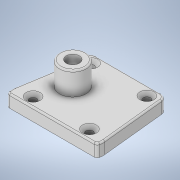
# Autodesk Inventor part: LegPin_Side_fillet_v1
Saved by Autodesk Inventor 2020.3 (Build 243373000, 373)
## iProperties
Created: 2021-03-02
Part Number: LegPin_Side_fillet_v1
Material: Generic
Document SubType Name: Modeling
Designer: sanyi
Density: 1 g/cm^3
Appearance: Default
Author: sanyi
Autodesk Inventor part; units mm, degrees
ref_plane "YZ Plane" through (0, 0, 0) normal (1, 0, 0) x (0, 1, 0)
ref_plane "XZ Plane" through (0, 0, 0) normal (0, 1, 0) x (-1, 0, 0)
ref_plane "XY Plane" through (0, 0, 0) normal (0, 0, 1) x (1, 0, 0)
sketch "Sketch1" plane through (0, 0, 0) normal (0, 1, 0) x (-1, 0, 0)
  line L0 (0, 114.579) -> (0, -115.31) construction
  line L1 (119.896, 0) -> (-136.2997, 0) construction
  line L2 (65, 45) -> (31.9074, 45) construction
  line L3 (-65, 45) -> (-65, 11.9074) construction
  line L4 (-65, -45) -> (-19.7, -45) construction
  line L5 (65, -45) -> (65, -11.9074) construction
  line L6 (64.9671, -36.1989) -> (82.3619, -53.5938) construction
  line L7 (82.3619, -53.5938) -> (73.5938, -62.3619) construction
  line L8 (73.5938, -62.3619) -> (56.1989, -44.9671) construction
  line L9 (56.1989, -44.9671) -> (64.9671, -36.1989) construction
  line L10 (64.9671, 36.1989) -> (82.3619, 53.5938) construction
  line L11 (82.3619, 53.5938) -> (73.5938, 62.3619) construction
  line L12 (73.5938, 62.3619) -> (56.1989, 44.9671) construction
  line L13 (56.1989, 44.9671) -> (64.9671, 36.1989) construction
  line L14 (-56.1989, 44.9671) -> (-73.5938, 62.3619) construction
  line L15 (-73.5938, 62.3619) -> (-82.3619, 53.5938) construction
  line L16 (-82.3619, 53.5938) -> (-64.9671, 36.1989) construction
  line L17 (-64.9671, 36.1989) -> (-56.1989, 44.9671) construction
  line L18 (-56.1989, -44.9671) -> (-73.5938, -62.3619) construction
  line L19 (-73.5938, -62.3619) -> (-82.3619, -53.5938) construction
  line L20 (-82.3619, -53.5938) -> (-64.9671, -36.1989) construction
  line L21 (-64.9671, -36.1989) -> (-56.1989, -44.9671) construction
  line L22 (55, 30) -> (-15, 30) construction
  line L23 (-15, 30) -> (-15, -30) construction
  line L24 (-15, -30) -> (55, -30) construction
  line L25 (55, -30) -> (55, 30) construction
  line L26 (73.6645, 44.8963) -> (64.8963, 53.6645) construction
  line L27 (68.7854, 57.5536) -> (77.5536, 48.7854) construction
  circle A0 centre (73.1695, 53.1695) radius 4.25 construction
  line L28 (73.6645, -44.8963) -> (64.8963, -53.6645) construction
  line L29 (77.5536, -48.7854) -> (68.7854, -57.5536) construction
  circle A1 centre (73.1695, -53.1695) radius 4.25 construction
  line L30 (-64.8963, 53.6645) -> (-73.6645, 44.8963) construction
  line L31 (-68.7854, 57.5536) -> (-77.5536, 48.7854) construction
  circle A2 centre (-73.1695, 53.1695) radius 4.25 construction
  line L32 (-73.6645, -44.8963) -> (-64.8963, -53.6645) construction
  line L33 (-77.5536, -48.7854) -> (-68.7854, -57.5536) construction
  circle A3 centre (-73.1695, -53.1695) radius 4.25 construction
  line L34 (6.8, 51.2) -> (-17.8, 51.2)
  line L35 (-17.8, 51.2) -> (-17.8, 38.8)
  line L36 (-17.8, 38.8) -> (6.8, 38.8)
  line L37 (6.8, 38.8) -> (6.8, 51.2)
  line L38 (6.8, -38.8) -> (-17.8, -38.8) construction
  line L39 (-17.8, -38.8) -> (-17.8, -51.2) construction
  line L40 (-17.8, -51.2) -> (6.8, -51.2) construction
  line L41 (6.8, -51.2) -> (6.8, -38.8) construction
  line L42 (6.8, 45) -> (-17.8, 45) construction
  line L43 (-5.5, 51.2) -> (-5.5, 38.8) construction
  line L44 (0, 51.2) -> (0, 38.8) construction
  line L45 (6.8, -45) -> (-17.8, -45) construction
  line L46 (-5.5, -38.8) -> (-5.5, -51.2) construction
  line L47 (0, -38.8) -> (0, -51.2) construction
  circle A4 centre (0, 45) radius 4.25
  circle A5 centre (0, -45) radius 4.25 construction
  line L48 (20, 30) -> (20, -30) construction
  line L49 (8.8, 57.2) -> (-19.8, 57.2)
  line L50 (8.8, -57.2) -> (-19.8, -57.2) construction
  line L51 (8.8, 57.2) -> (8.8, 45) construction
  line L52 (-19.8, 57.2) -> (-19.8, 45) construction
  line L53 (8.8, -57.2) -> (8.8, -45) construction
  line L54 (-19.8, -57.2) -> (-19.8, -45) construction
  line L55 (67.2298, 63.069) -> (61.3608, 57.2) construction
  line L56 (83.069, 47.2298) -> (77.2, 41.3608) construction
  line L57 (64.8963, 53.6645) -> (61.3608, 57.2) construction
  line L58 (73.6645, 44.8963) -> (77.2, 41.3608) construction
  arc A6 (83.069, 47.2298) -> (67.2298, 63.069) centre (75.1494, 55.1494) ccw construction
  line L59 (-61.3608, 57.2) -> (-67.2298, 63.069) construction
  line L60 (-83.069, 47.2298) -> (-77.2, 41.3608) construction
  line L61 (-61.3608, 57.2) -> (-64.8963, 53.6645) construction
  line L62 (-77.2, 41.3608) -> (-73.6645, 44.8963) construction
  arc A7 (-67.2298, 63.069) -> (-83.069, 47.2298) centre (-75.1494, 55.1494) ccw construction
  line L63 (73.6645, -44.8963) -> (77.2, -41.3608) construction
  line L64 (77.2, -41.3608) -> (83.069, -47.2298) construction
  line L65 (64.8963, -53.6645) -> (61.3608, -57.2) construction
  line L66 (61.3608, -57.2) -> (67.2298, -63.069) construction
  arc A8 (67.2298, -63.069) -> (83.069, -47.2298) centre (75.1494, -55.1494) ccw construction
  line L67 (-73.6645, -44.8963) -> (-77.2, -41.3608) construction
  line L68 (-64.8963, -53.6645) -> (-61.3608, -57.2) construction
  line L69 (-61.3608, -57.2) -> (-67.2298, -63.069) construction
  line L70 (-77.2, -41.3608) -> (-83.069, -47.2298) construction
  arc A9 (-83.069, -47.2298) -> (-67.2298, -63.069) centre (-75.1494, -55.1494) ccw construction
  arc A10 (23.5363, -45) -> (8.8, -57.2) centre (23.5363, -60) ccw construction
  arc A11 (61.3608, -57.2) -> (31.9074, -45) centre (31.9074, -86.6534) ccw construction
  arc A12 (65, -11.9074) -> (77.2, -41.3608) centre (106.6534, -11.9074) ccw construction
  arc A13 (77.2, 41.3608) -> (65, 11.9074) centre (106.6534, 11.9074) ccw construction
  arc A14 (31.9074, 45) -> (61.3608, 57.2) centre (31.9074, 86.6534) ccw construction
  arc A15 (8.8, 57.2) -> (23.5363, 45) centre (23.5363, 60) ccw
  arc A16 (-65, 11.9074) -> (-77.2, 41.3608) centre (-106.6534, 11.9074) ccw construction
  arc A17 (-77.2, -41.3608) -> (-65, -11.9074) centre (-106.6534, -11.9074) ccw construction
  line L71 (73.1695, -53.1695) -> (-73.1695, -53.1695) construction
  line L72 (-73.1695, 53.1695) -> (73.1695, 53.1695) construction
  line L73 (-61.3608, 57.2) -> (-61.3608, 45) construction
  line L74 (-61.3608, -57.2) -> (-61.3608, -45) construction
  arc A18 (-19.8, -57.2) -> (-34.5363, -45) centre (-34.5363, -60) ccw construction
  arc A19 (-31.9074, -45) -> (-61.3608, -57.2) centre (-31.9074, -86.6534) ccw construction
  arc A20 (-34.5363, 45) -> (-33.5506, 45.0324) centre (-34.5363, 60) ccw
  arc A21 (-61.3608, 57.2) -> (-33.5506, 45.0324) centre (-31.9074, 86.6534) ccw construction
  line L75 (73.5938, 62.3619) -> (76.4222, 65.1903) construction
  line L76 (76.4222, 65.1903) -> (85.1903, 56.4222) construction
  line L77 (85.1903, 56.4222) -> (82.3619, 53.5938) construction
  line L78 (79.3213, 59.3213) -> (59.2395, 39.2395) construction
  line L79 (59.2395, -39.2395) -> (79.3213, -59.3213) construction
  line L80 (-79.3213, 59.3213) -> (-59.2395, 39.2395) construction
  line L81 (-79.3213, -59.3213) -> (-59.2395, -39.2395) construction
  line L82 (75.1494, 55.1494) -> (77.9778, 57.9778) construction
  line L83 (75.1494, -55.1494) -> (77.9778, -57.9778) construction
  line L84 (-75.1494, -55.1494) -> (-77.9778, -57.9778) construction
  line L85 (-75.1494, 55.1494) -> (-77.9778, 57.9778) construction
  line L86 (-19.7, 45) -> (-65, 45) construction
  line L87 (8.7, 45) -> (-19.7, 45) construction
  line L88 (8.7, -45) -> (23.5363, -45) construction
  line L89 (-19.7, -45) -> (8.7, -45) construction
  line L90 (82.3619, 53.5938) -> (85.3751, 50.5805) construction
  line L91 (73.5938, 62.3619) -> (70.5805, 65.3751) construction
  line L92 (80.1698, 55.7858) -> (75.3615, 50.9775) construction
  line L93 (70.9775, -55.3615) -> (75.7858, -60.1698) construction
  line L94 (0, -48.1) -> (6.8, -48.1) construction
  line L95 (-75.3615, -50.9775) -> (-80.1698, -55.7858) construction
  line L96 (-75.7858, 60.1698) -> (-70.9775, 55.3615) construction
  line L97 (0, 48.1) -> (6.8, 48.1) construction
  line L98 (82.3619, -53.5938) -> (85.3751, -50.5805) construction
  line L99 (73.5938, -62.3619) -> (70.5805, -65.3751) construction
  line L100 (-73.5938, -62.3619) -> (-70.5805, -65.3751) construction
  line L101 (-82.3619, -53.5938) -> (-85.3751, -50.5805) construction
  line L102 (-73.5938, 62.3619) -> (-70.5805, 65.3751) construction
  line L103 (-82.3619, 53.5938) -> (-85.3751, 50.5805) construction
  line L104 (31.9074, 45) -> (23.5363, 45) construction
  line L105 (23.5363, 45) -> (8.7, 45) construction
  arc A22 (-33.5506, 45.0324) -> (-31.9074, 45) centre (-31.9074, 86.6534) ccw
  arc A23 (-33.5506, 45.0324) -> (-19.8, 57.2) centre (-34.5363, 60) ccw
  line L106 (-21.9995, 42) -> (-51.9995, 42) construction
  line L107 (-51.9995, 42) -> (-51.9995, -42) construction
  line L108 (-51.9995, -42) -> (-21.9995, -42) construction
  line L109 (-21.9995, -42) -> (-21.9995, 42) construction
  line L110 (52, 27) -> (55, 27) construction
  line L111 (52, -27) -> (55, -27) construction
  line L112 (52, 27) -> (52, 30) construction
  line L113 (-12, 27) -> (-12, 30) construction
  line L114 (-12, 27) -> (-15, 27) construction
  line L115 (-15, -27) -> (-12, -27) construction
  line L116 (-12, -27) -> (-12, -30) construction
  line L117 (52, -27) -> (52, -30) construction
  line L118 (-19.4995, 10) -> (-20.9995, 10) construction
  line L119 (-20.9995, 10) -> (-20.9995, -10) construction
  line L120 (-20.9995, -10) -> (-19.4995, -10) construction
  line L121 (-19.4995, -10) -> (-19.4995, 10) construction
  line L122 (-19.4995, 0) -> (-20.9995, 0) construction
  line L123 (-36.9995, 42) -> (-36.9995, -42) construction
  line L124 (-52.9995, 10) -> (-54.4995, 10) construction
  line L125 (-54.4995, 10) -> (-54.4995, -10) construction
  line L126 (-54.4995, -10) -> (-52.9995, -10) construction
  line L127 (-52.9995, -10) -> (-52.9995, 10) construction
  line L128 (-52.9995, 0) -> (-54.4995, 0) construction
  line L129 (31.9074, -45) -> (65, -45) construction
  line L130 (23.5363, -45) -> (31.9074, -45) construction
  line L131 (65, -11.9074) -> (65, 11.9074) construction
  line L132 (65, 11.9074) -> (65, 45) construction
  arc A24 (68.1707, 27.8475) -> (64.9671, 36.1989) centre (57.1958, 28.4277) ccw construction
  arc A25 (56.1989, 44.9671) -> (47.8475, 48.1707) centre (48.4277, 37.1958) ccw construction
  arc A26 (64.9671, -36.1989) -> (68.1707, -27.8475) centre (57.1958, -28.4277) ccw construction
  arc A27 (47.8475, -48.1707) -> (56.1989, -44.9671) centre (48.4277, -37.1958) ccw construction
  arc A28 (-56.1989, -44.9671) -> (-47.8475, -48.1707) centre (-48.4277, -37.1958) ccw construction
  arc A29 (-68.1707, -27.8475) -> (-64.9671, -36.1989) centre (-57.1958, -28.4277) ccw construction
  arc A30 (-48.6036, 48.4926) -> (-56.1989, 44.9671) centre (-47.5843, 36.3524) ccw construction
  arc A31 (-64.9671, 36.1989) -> (-68.1707, 27.8475) centre (-57.1958, 28.4277) ccw construction
  line L133 (-65, 11.9074) -> (-65, -11.9074) construction
  line L134 (-65, -11.9074) -> (-65, -45) construction
  line L135 (-56.1989, 44.9671) -> (-56.1989, -44.9671) construction
  arc A32 (-19.9504, 56.5) -> (-17.8, 51.2) centre (-15.1706, 55.3531) ccw
  arc A33 (6.8, 51.2) -> (8.9504, 56.5) centre (4.1706, 55.3531) ccw
  arc A34 (8.9504, -56.5) -> (6.8, -51.2) centre (4.1706, -55.3531) ccw construction
  arc A35 (-17.8, -51.2) -> (-19.9504, -56.5) centre (-15.1706, -55.3531) ccw construction
  line L136 (-17.8, 38.8) -> (-17.8, 32.8)
  line L137 (-17.8, 32.8) -> (6.8, 32.8)
  line L138 (6.8, 32.8) -> (6.8, 38.8)
  line L139 (-17.8, -38.8) -> (-17.8, -32.8) construction
  line L140 (-17.8, -32.8) -> (6.8, -32.8) construction
  line L141 (6.8, -32.8) -> (6.8, -38.8) construction
  line L142 (3.5, 54.2) -> (3.5, 35.8) construction
  line L143 (3.5, 35.8) -> (-14.5, 35.8) construction
  line L144 (-14.5, 35.8) -> (-14.5, 54.2) construction
  line L145 (-14.5, 54.2) -> (3.5, 54.2) construction
  line L146 (9.0232, 54.5696) -> (6.8, 40.8)
  line L147 (-20.0605, 54.8518) -> (-17.8, 32.8)
  point P0 (0, 0)
  point P1 (64.9853, 0)
  point P2 (55, 0)
  point P3 (60.583, -40.583)
  point P4 (-59.2395, 39.2395)
  point P5 (-60.583, 40.583)
  point P6 (-60.583, -40.583)
  point P7 (0, 45)
  point P8 (-33.9298, 45.0048)
  point P9 (-33.5506, -45.0324)
  point P10 (-56.1658, -45)
  point P11 (-56.2319, -45)
  point P12 (-56.2319, 45)
  point P13 (-56.1659, 45)
  point P14 (-20.0537, 54.7901)
  point P15 (6.8, 33.8)
  dimension "d0" = 135
  dimension "d4" = 24.6
  dimension "d5" = 12.4
  dimension "d6" = 70
  dimension "d7" = 60
  dimension "d9" = 8.5
  dimension "d10" = 135
  dimension "d12" = 6
  dimension "d13" = 2
  dimension "d14" = 2
  dimension "d16" = 20
  dimension "d23" = 5
  dimension "d29" = 130
  dimension "d32" = 15
  dimension "d33" = 4
  dimension "d34" = 28.4
  dimension "d38" = 4
  dimension "d40" = 6.8
  dimension "d49" = 30
  dimension "d50" = 84
  dimension "d51" = 3
  dimension "d52" = 3
  dimension "d53" = 1.5
  dimension "d54" = 20
  dimension "d59" = 1
  dimension "d60" = 90
  dimension "d61" = 135
  dimension "d70" = 135
  dimension "d82" = 0.7
  dimension "d83" = 0.7
  dimension "d84" = 0.7
  dimension "d85" = 0.7
  dimension "d86" = 6
  dimension "d102" = 18
  dimension "d126" = 2
  constraints: 294 end point, 89 tangent, 83 point on circle, 82 point on line, 80 perpendicular, 67 parallel, 42 midpoint, 40 equal length, 36 centre point, 18 horizontal, 15 collinear, 10 coincident, 8 equal radius, 7 symmetric about line, 3 vertical, 33 other
  measures "d0" angle of L3 L16
  measures "d4" distance between parallel lines of L11 L13
  measures "d5" distance between parallel lines of L10 L12
  measures "d6" distance of L24.end L23.end
  measures "d7" distance of L23.end L22.end
  measures "d9" diameter of A0
  measures "d10" angle of L6 L5
  measures "d12" distance between parallel lines of L34 L49
  measures "d13" distance between parallel lines of L37 L51
  measures "d14" distance between parallel lines of L41 L53
  measures "d16" distance between parallel lines of L0 L48
  measures "d23" distance between parallel lines of L56 L10
  measures "d29" distance between parallel lines of L3 L5
  measures "d32" radius of A15
  measures "d33" distance between parallel lines of L76 L11
  measures "d34" distance of L78.start L78.end
  measures "d38" distance of L82.start L82.end
  measures "d40" distance between parallel lines of L11 L27
  measures "d49" distance of L108.end L107.end
  measures "d50" distance of L107.end L106.end
  measures "d51" distance of L110.start L110.end
  measures "d52" distance of L110.start L112.end
  measures "d53" distance of L120.end L119.end
  measures "d54" distance of L119.end L118.end
  measures "d59" distance between parallel lines of L109 L119
  measures "d60" distance between parallel lines of L2 L88
  measures "d61" angle of L132 L10
  measures "d70" angle of L134 L20
  measures "d82" vertical distance of L49.end A32.start
  measures "d83" vertical distance of L49.start A33.end
  measures "d84" vertical distance of L50.start A34.start
  measures "d85" vertical distance of L50.end A35.end
  measures "d86" distance between parallel lines of L36 L137
  measures "d102" distance of L142.end L143.end
  measures "d126" distance from line of L36 L146.end
extrude "Extrusion12" add sketch "Sketch1" along normal blind 4 contours A33 L146 L37 | L34 A32 A23 L49 A15 A33 | L35 L136 L147 A32 | L36 L138 L137 L136
extrude "Extrusion13" add sketch "Sketch1" along normal blind 4 contours L37 L36 L35 L34
extrude "Extrusion14" add sketch "Sketch1" along normal blind 11.4 contours A4
sketch "Sketch2" plane through (0, 11.4, 45) normal (0, 1, 0) x (1, 0, 0)
  point P0 (0, 45)
  point P1 (0, 0)
hole "Hole3" at (0, 11.4, 45) direction (0, -1, 0) diameter 4.2 end through all
fillet "Fillet10" radius 2 2 edges at (-6.8, 2, 32.8) (17.8, 2, 32.8)
fillet "Fillet10" radius 1 2 edges at (19.8, 2, 57.2) (-8.8, 2, 57.2)
fillet "Fillet11" radius 0.5 11 edges at (19.6194, 4, 56.9798) (20.0778, 4, 55.6377) (-8.6194, 4, 56.9798) (-9.084, 4, 55.4955) (5.5, 4, 57.2) (5.5973, 4, 32.8) (4.25, 11.4, 45) (19.0223, 4, 44.7239) (17.3347, 4, 33.3154) (-6.2142, 4, 33.3858) (-7.9116, 4, 47.6848)
sketch "Sketch4" plane through (0, 4, 0) normal (0, 1, 0) x (1, 0, 0)
  point P0 (0, 0)
  point P1 (-3.5, -54.2)
  point P2 (14.5, -54.2)
  point P3 (14.5, -35.8)
  point P4 (-3.5, -35.8)
hole "Hole4" at (-3.5, 4, 54.2) at (-3.5, 4, 35.8) at (14.5, 4, 35.8) at (14.5, 4, 54.2) direction (0, -1, 0) diameter 2.3 depth 6.5 countersink diameter 4.5 countersink angle 90
hole "Hole5" at (0, 0, 45) direction (0, 1, 0) diameter 5.6 depth 6.5 counterbore diameter 9 counterbore depth 1
body "Solid6"
